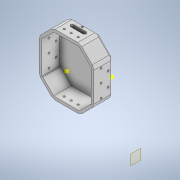
# Autodesk Inventor part: magnetbox
Saved by Autodesk Inventor 2022 (Build 260153000, 153)
## iProperties
Created: 2023-03-07
Part Number: magnetbox
Material: Generic
Document SubType Name: Modeling
Designer: chris
Density: 1 g/cm^3
Appearance: Default
Author: chris
Autodesk Inventor part; units mm, degrees
ref_plane "YZ Plane" through (0, 0, 0) normal (1, 0, 0) x (0, 1, 0)
ref_plane "XZ Plane" through (0, 0, 0) normal (0, 1, 0) x (-1, 0, 0)
ref_plane "XY Plane" through (0, 0, 0) normal (0, 0, 1) x (1, 0, 0)
sketch "Sketch1" plane through (0, 0, 0) normal (0, 0, 1) x (1, 0, 0)
  line L0 (-53, -34) -> (-53, 34)
  line L1 (-59, 36.4853) -> (-59, -36.4853)
  line L2 (-29.4853, -66) -> (29.4853, -66)
  line L3 (51, -36) -> (27.5, -59.5)
  line L4 (51, -36) -> (27.5, -59.5)
  line L5 (44.2426, -51.2426) -> (29.4853, -66)
  line L6 (44.2426, -51.2426) -> (59, -36.4853)
  line L7 (51, 36) -> (27.5, 59.5)
  line L8 (51, 36) -> (27.5, 59.5)
  line L9 (44.2426, 51.2426) -> (29.4853, 66)
  line L10 (44.2426, 51.2426) -> (59, 36.4853)
  line L11 (-51, -36) -> (-27.5, -59.5)
  line L12 (-51, -36) -> (-27.5, -59.5)
  line L13 (-44.2426, -51.2426) -> (-29.4853, -66)
  line L14 (-44.2426, -51.2426) -> (-59, -36.4853)
  line L15 (-44.2426, 51.2426) -> (-59, 36.4853)
  line L16 (-51, 36) -> (-27.5, 59.5)
  line L17 (-44.2426, 51.2426) -> (-29.4853, 66)
  line L18 (59, -36.4853) -> (59, 36.4853)
  line L19 (53, 34) -> (53, -34)
  line L20 (-29.4853, 66) -> (29.4853, 66)
  line L21 (0, 59.5) -> (-27.5, 59.5)
  line L22 (0, 59.5) -> (27.5, 59.5)
  line L23 (59, 0) -> (75.3733, 0)
  line L24 (0, -59.5) -> (-27.5, -59.5)
  line L25 (0, -59.5) -> (27.5, -59.5)
  line L26 (-53, 0) -> (53, 0)
  line L27 (-53, -34) -> (-53, -36)
  line L28 (-53, -36) -> (-51, -36)
  line L29 (-53, 34) -> (-53, 36)
  line L30 (-53, 36) -> (-51, 36)
  line L31 (53, 34) -> (53, 36)
  line L32 (53, 36) -> (51, 36)
  line L33 (53, -34) -> (53, -36)
  line L34 (53, -36) -> (51, -36)
  point P0 (-35.4853, -60)
  dimension "d56" = 2
  dimension "d57" = 2
  dimension "d58" = 2
  constraints: 70 end point, 5 vertical, 4 perpendicular, 3 horizontal, 3 midpoint, 3 symmetric about line, 1 point on line
  measures "d56" distance of L0.start L27.end
  measures "d57" distance of L0.end L29.end
  measures "d58" distance of L19.end L33.end
extrude "Extrusion1" add sketch "Sketch1" along normal blind 38
sketch "Sketch2" plane through (0, 0, 0) normal (0, 0, -1) x (-1, 0, 0)
  line L0 (29.4853, -66) -> (-29.4853, -66) projected
  line L1 (59, 36.4853) -> (59, -36.4853) projected
  line L2 (-59, 36.4853) -> (-29.4853, 66) projected
  line L3 (-59, -36.4853) -> (-59, 36.4853) projected
  line L4 (-29.4853, -66) -> (-59, -36.4853) projected
  line L5 (59, -36.4853) -> (29.4853, -66) projected
  line L6 (29.4853, 66) -> (59, 36.4853) projected
  line L7 (-29.4853, 66) -> (29.4853, 66) projected
  point P0 (0, 0)
extrude "Extrusion2" add sketch "Sketch2" along normal blind 3
ref_plane "Work Plane1" through (112, -122, 1) normal (1, 0, 0) x (0, 0, -1)
sketch "Sketch7" plane through (59, -36.4853, 38) normal (1, 0, 0) x (0, 0, -1)
  circle A0 centre (30.2642, 51.6031) radius 2
  circle A1 centre (30.2642, 21.3675) radius 2
  circle A2 centre (15, 64.4853) radius 2
  circle A3 centre (15, 36.4853) radius 2
  circle A4 centre (15, 8.4853) radius 2
  line L0 (0, 0.4853) -> (0, 72.4853) projected
  line L1 (0, 36.4853) -> (15, 36.4853)
  point P0 (38, 36.4853)
  point P1 (0, 2.4853)
  point P2 (0, 70.4853)
  dimension "d17" = 4
  dimension "d18" = 4
  dimension "d19" = 15
  constraints: 5 centre point, 2 end point, 1 horizontal, 1 midpoint
  measures "d17" diameter of A1
  measures "d18" diameter of A3
  measures "d19" distance of L1.start L1.end
extrude "Extrusion4" cut sketch "Sketch7" against normal through all
chamfer "Chamfer1" distance 5 angle 45 8 edges at (29.4853, 66, 17.5) (59, 36.4853, 17.5) (-29.4853, 66, 17.5) (-59, 36.4853, 17.5) (59, -36.4853, 17.5) (29.4853, -66, 17.5) (-29.4853, -66, 17.5) (-59, -36.4853, 17.5)
chamfer "Chamfer2" distance 5 angle 45 8 edges at (44.2426, 51.2426, -3) (-44.2426, 51.2426, -3) (0, 66, -3) (-59, 0, -3) (-44.2426, -51.2426, -3) (59, 0, -3) (44.2426, -51.2426, -3) (0, -66, -3)
sketch "Sketch8" plane through (-24.4853, 66, 38) normal (0, 1, 0) x (1, 0, 0)
  line L0 (48.9706, 36) -> (0, 36) projected
  line L1 (26.4278, 21.2661) -> (42.4278, 21.2661)
  line L2 (42.4278, 21.2661) -> (42.4278, 28.6949)
  line L3 (42.4278, 28.6949) -> (7.4278, 28.6949)
  line L4 (7.4278, 28.6949) -> (7.4278, 21.2661)
  line L5 (7.4278, 21.2661) -> (26.4278, 21.2661)
  line L6 (7.4278, 24.9805) -> (11.1422, 28.6949)
  line L7 (7.4278, 24.9805) -> (12.6807, 24.9805) construction
  line L8 (24.9278, 28.6949) -> (24.9278, 33.6553)
  line L9 (7.4278, 24.9805) -> (4.6752, 24.9805)
  line L10 (7.4278, 24.9805) -> (11.1422, 21.2661)
  line L11 (42.4278, 24.9805) -> (38.7134, 28.6949)
  line L12 (42.4278, 24.9805) -> (38.7134, 21.2661)
  circle A0 centre (24.9278, 33.6553) radius 2
  point P0 (24.4853, 38)
  point P1 (38.7134, 21.2661)
  dimension "d30" = 16
  dimension "d31" = 35
  dimension "d32" = 45
  dimension "d59" = 4
  constraints: 24 end point, 4 symmetric about line, 3 perpendicular, 3 point on line, 2 horizontal, 2 midpoint, 1 centre point, 1 coincident, 1 equal length, 1 vertical
  measures "d30" distance of L1.start L1.end
  measures "d31" distance of L2.end L3.end
  measures "d32" angle of L7 L6
  measures "d59" diameter of A0
extrude "Extrusion5" cut sketch "Sketch8" against normal blind 10 contours L5 L10 L6 L3 L11 L12 L1 | A0
sketch "Sketch9" plane through (-24.4853, 66, 38) normal (0, 1, 0) x (1, 0, 0)
  line L0 (-3.0147, 0) -> (51.9853, 0) projected
  line L1 (24.4853, 0) -> (24.4853, 10)
  line L2 (24.4853, 10) -> (9.4853, 10)
  line L3 (9.4853, 10) -> (39.4853, 10)
  circle A0 centre (24.4853, 10) radius 2
  circle A1 centre (39.4853, 10) radius 2
  circle A2 centre (9.4853, 10) radius 2
  point P0 (24.4853, 38)
  dimension "d35" = 10
  dimension "d36" = 15
  dimension "d37" = 30
  dimension "d38" = 4
  dimension "d39" = 4
  dimension "d40" = 4
  constraints: 6 end point, 3 centre point, 3 coincident, 1 midpoint, 1 perpendicular, 1 point on line, 1 vertical
  measures "d35" distance of L1.start L1.end
  measures "d36" distance of L1.end L2.end
  measures "d37" distance of L2.end L3.end
  measures "d38" diameter of A0
  measures "d39" diameter of A1
  measures "d40" diameter of A2
extrude "Extrusion6" cut sketch "Sketch9" against normal through all
sketch "Sketch10" plane through (0, 0, -3) normal (0, 0, -1) x (-1, 0, 0)
  arc A0 (36.5359, -2) -> (36.5359, 2) centre (40, 0) ccw
  arc A1 (-36.5359, 2) -> (-36.5359, -2) centre (-40, 0) ccw
  line L0 (36.5359, -2) -> (7.746, -2)
  line L1 (-7.746, -2) -> (-36.5359, -2)
  line L2 (20, 16.2488) -> (20, 11.2488)
  arc A2 (20, 16.2488) -> (-20, 16.2488) centre (0, -10) ccw
  arc A3 (20, 11.2488) -> (-20, 11.2488) centre (0, -15) ccw
  line L3 (-20, 16.2488) -> (-20, 11.2488)
  line L4 (22, 29.006) -> (22, 39.387)
  arc A4 (22, 29.006) -> (-22, 29.006) centre (0, 7.1657) ccw
  arc A5 (22, 39.387) -> (-22, 39.387) centre (0, 12.1657) ccw
  line L5 (-22, 39.387) -> (-22, 29.006)
  arc A6 (-22, -39.387) -> (22, -39.387) centre (0, -12.1657) ccw
  line L6 (22, -29.006) -> (22, -39.387)
  arc A7 (-22, -29.006) -> (22, -29.006) centre (0, -7.1657) ccw
  arc A8 (-20, -16.2488) -> (20, -16.2488) centre (0, 10) ccw
  line L7 (20, -16.2488) -> (20, -11.2488)
  arc A9 (-20, -11.2488) -> (20, -11.2488) centre (0, 15) ccw
  line L8 (-22, -39.387) -> (-22, -29.006)
  line L9 (-20, -16.2488) -> (-20, -11.2488)
  line L10 (36.5359, 2) -> (7.746, 2)
  line L11 (-7.746, 2) -> (-36.5359, 2)
  arc A10 (-7.746, -2) -> (7.746, -2) centre (0, 0) ccw
  arc A11 (7.746, 2) -> (-7.746, 2) centre (0, 0) ccw
  line L12 (0, -15) -> (-12.9904, -7.5)
  line L13 (-12.9904, -7.5) -> (-12.9904, 7.5)
  line L14 (-12.9904, 7.5) -> (0, 15)
  line L15 (0, 15) -> (12.9904, 7.5)
  line L16 (12.9904, 7.5) -> (12.9904, -7.5)
  line L17 (12.9904, -7.5) -> (0, -15)
  point P0 (0, -2)
  point P1 (-40, -2)
  point P2 (0, 2)
  point P3 (-40, 2)
  point P4 (-12.9904, -2)
  point P5 (12.9904, -2)
  point P6 (12.9904, 2)
  point P7 (-12.9904, 2)
  dimension "d44" = 8
  dimension "d45" = 8
  constraints: 36 end point, 24 point on circle, 12 centre point, 2 vertical, 1 coincident, 13 other
  measures "d44" diameter of A0
  measures "d45" diameter of A1
extrude "Extrusion7" cut sketch "Sketch10" against normal blind 0.25 contours L0 L16 L10 A0 | L0 A10 L1 L13 L11 A11 L10 L16 | L1 A1 L11 L13 | L2 A3 L3 A2 | A4 L5 A5 L4 | L8 A7 L6 A6 | L9 A9 L7 A8
extrude "Extrusion8" cut sketch "Sketch10" against normal blind 0.5 contours L16 L17 L12 L13 L1 A10 L0 | L10 A11 L11 L13 L14 L15 L16
sketch "Sketch11" plane through (0, 0, -2.75) normal (0, 0, -1) x (-1, 0, 0)
  line L0 (-7.746, -2) -> (-12.9904, -2) projected
  arc A0 (-7.746, -2) -> (7.746, -2) centre (0, 0) ccw projected
  line L1 (12.9904, -2) -> (7.746, -2) projected
  line L2 (36.5359, -2) -> (12.9904, -2) projected
  arc A1 (36.5359, -2) -> (36.5359, 2) centre (40, 0) ccw projected
  line L3 (12.9904, 2) -> (36.5359, 2) projected
  line L4 (7.746, 2) -> (12.9904, 2) projected
  arc A2 (7.746, 2) -> (-7.746, 2) centre (0, 0) ccw projected
  line L5 (-12.9904, 2) -> (-7.746, 2) projected
  line L6 (-36.5359, 2) -> (-12.9904, 2) projected
  arc A3 (-36.5359, 2) -> (-36.5359, -2) centre (-40, 0) ccw projected
  line L7 (-12.9904, -2) -> (-36.5359, -2) projected
  line L8 (12.9904, 7.5) -> (12.9904, 2) projected
  line L9 (36.5359, -2) -> (12.9904, -2) projected
  line L10 (12.9904, 2) -> (12.9904, -2)
  line L11 (-12.9904, 2) -> (-12.9904, 7.5) projected
  line L12 (-12.9904, -2) -> (-7.746, -2) projected
  line L13 (-12.9904, 2) -> (-12.9904, -2)
  constraints: 4 end point, 2 vertical
extrude "Extrusion9" add sketch "Sketch11" along normal up to surface (0.25 mm away) contours L0 L13 L5 A2 L4 L10 L1 A0
sketch "Sketch14" plane through (0, 0, 38) normal (0, 0, 1) x (1, 0, 0)
  point P0 (0, 0)
sketch "Sketch15" plane through (59, -31.4853, 38) normal (1, 0, 0) x (0, 0, -1)
  point P0 (38, 31.4853)
body "Solid1"
